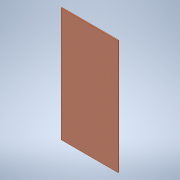
# Autodesk Inventor part: madera
Saved by Autodesk Inventor 2021 (Build 250183000, 183)
## iProperties
Created: 2023-12-09
Part Number: madera
Material: Generic
Document SubType Name: Modeling
Designer: assman
Density: 1 g/cm^3
Appearance: Walnut - Natural Polished
Author: assman
Autodesk Inventor part; units mm, degrees
ref_plane "YZ Plane" through (0, 0, 0) normal (1, 0, 0) x (0, 1, 0)
ref_plane "XZ Plane" through (0, 0, 0) normal (0, 1, 0) x (-1, 0, 0)
ref_plane "XY Plane" through (0, 0, 0) normal (0, 0, 1) x (1, 0, 0)
sketch "Sketch1" plane through (0, 0, 0) normal (0, 0, 1) x (1, 0, 0)
  line L0 (-625, 1250) -> (625, 1250)
  line L1 (625, 1250) -> (625, -1250)
  line L2 (625, -1250) -> (-625, -1250)
  line L3 (-625, -1250) -> (-625, 1250)
  line L4 (-625, 1250) -> (625, -1250) construction
  line L5 (625, 1250) -> (-625, -1250) construction
  point P0 (0, 0)
  dimension "d0" = 1250
  dimension "d1" = 2500
  constraints: 12 end point, 2 midpoint, 2 parallel, 1 horizontal, 1 perpendicular
  measures "d0" distance of L1.end L2.end
  measures "d1" distance of L0.end L1.end
extrude "Extrusion1" add sketch "Sketch1" along normal blind 20
body "Solid1"
